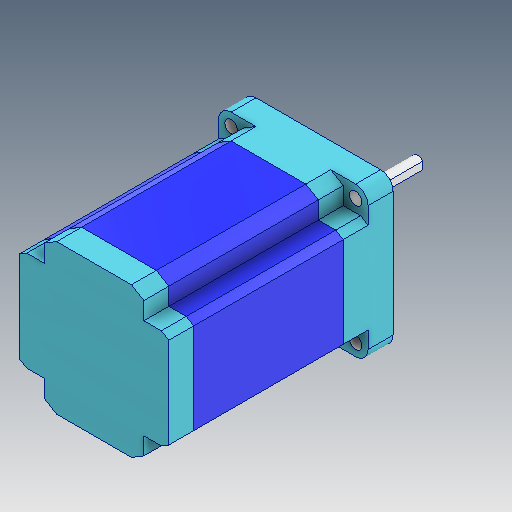
# Autodesk Inventor part: servo
Saved by Autodesk Inventor 2021 (Build 250183000, 183)
## iProperties
Created: 2021-07-07
Part Number: servo
Material: Generic
Document SubType Name: Modeling
Designer: Shaheen Khan
Density: 1 g/cm^3
Appearance: Aluminum - Flat
Author: Shaheen Khan
Autodesk Inventor part; units mm, degrees
ref_plane "XZ Plane" through (0, 0, 0) normal (0, 1, 0) x (-1, 0, 0)
ref_plane "XY Plane" through (0, 0, 0) normal (0, 0, 1) x (1, 0, 0)
sketch "Sketch1" plane through (0, 0, 0) normal (0, 0, 1) x (1, 0, 0)
  line L0 (-30, 30) -> (30, 30)
  line L1 (30, 30) -> (30, -30)
  line L2 (30, -30) -> (-30, -30)
  line L3 (-30, -30) -> (-30, 30)
  line L4 (-30, 30) -> (30, -30) construction
  line L5 (30, 30) -> (-30, -30) construction
  point P0 (0, 0)
  dimension "d0" = 60
  dimension "d1" = 60
  constraints: 12 end point, 2 midpoint, 2 parallel, 1 horizontal, 1 perpendicular
  measures "d0" distance of L1.end L2.end
  measures "d1" distance of L0.end L1.end
extrude "Extrusion1" add sketch "Sketch1" along normal blind 10
sketch "Sketch2" plane through (0, 0, 10) normal (0, 0, 1) x (1, 0, 0)
  line L0 (-30, -30) -> (30, -30) projected
  line L1 (30, -30) -> (30, 30) projected
  line L2 (30, 30) -> (-30, 30) projected
  line L3 (-30, 30) -> (-30, -30) projected
  line L4 (30, 30) -> (-30, 30) projected
  line L5 (0, 30) -> (-15, 30)
  line L6 (-15, 30) -> (-20, 27)
  line L7 (-20, 27) -> (-20, 20)
  line L8 (-20, 20) -> (-27, 20)
  line L9 (-27, 20) -> (-30, 18.2)
  line L10 (-30, 30) -> (-30, -30) projected
  line L11 (0, 30) -> (0, 0)
  line L12 (0, 0) -> (-30, 0)
  line L13 (15, 30) -> (20, 27)
  line L14 (20, 27) -> (20, 20)
  line L15 (20, 20) -> (27, 20)
  line L16 (27, 20) -> (30, 18.2)
  line L17 (0, -30) -> (-15, -30)
  line L18 (-15, -30) -> (-20, -27)
  line L19 (-20, -27) -> (-20, -20)
  line L20 (-20, -20) -> (-27, -20)
  line L21 (-27, -20) -> (-30, -18.2)
  line L22 (15, -30) -> (20, -27)
  line L23 (20, -27) -> (20, -20)
  line L24 (20, -20) -> (27, -20)
  line L25 (27, -20) -> (30, -18.2)
  dimension "d4" = 15
  dimension "d5" = 3
  dimension "d6" = 5
  dimension "d7" = 10
  dimension "d8" = 3
  constraints: 40 end point, 16 symmetric about line, 2 midpoint, 2 perpendicular, 2 point on line, 1 parallel
  measures "d4" distance of L5.start L5.end
  measures "d5" vertical distance of L6.end L5.end
  measures "d6" horizontal distance of L5.end L6.end
  measures "d7" distance between parallel lines of L8 L2
  measures "d8" horizontal distance of L8.end L9.end
extrude "Extrusion2" add sketch "Sketch2" along normal blind 10 contours L18 L19 L20 L21 L3 L12 L11 L2 L13 L14 L15 L16 L1 L25 L24 L23 L22 L0 | L3 L9 L8 L7 L6 L2 L11 L12
sketch "Sketch3" plane through (0, 0, 20) normal (0, 0, 1) x (1, 0, 0)
  line L0 (-27, 20) -> (-30, 18.2) projected
  line L1 (-30, 18.2) -> (-30, -18.2) projected
  line L2 (-30, -18.2) -> (-27, -20) projected
  line L3 (-27, -20) -> (-20, -20) projected
  line L4 (-20, -20) -> (-20, -27) projected
  line L5 (-20, -27) -> (-15, -30) projected
  line L6 (-15, -30) -> (15, -30) projected
  line L7 (15, -30) -> (20, -27) projected
  line L8 (20, -27) -> (20, -20) projected
  line L9 (20, -20) -> (27, -20) projected
  line L10 (27, -20) -> (30, -18.2) projected
  line L11 (30, -18.2) -> (30, 18.2) projected
  line L12 (30, 18.2) -> (27, 20) projected
  line L13 (27, 20) -> (20, 20) projected
  line L14 (20, 20) -> (20, 27) projected
  line L15 (20, 27) -> (15, 30) projected
  line L16 (15, 30) -> (-15, 30) projected
  line L17 (-15, 30) -> (-20, 27) projected
  line L18 (-20, 27) -> (-20, 20) projected
  line L19 (-20, 20) -> (-27, 20) projected
  point P0 (0, 0)
extrude "Extrusion3" add sketch "Sketch3" along normal blind 60 separate body
sketch "Sketch4" plane through (0, 0, 80) normal (0, 0, 1) x (1, 0, 0)
  line L0 (-30, 18.2) -> (-30, -18.2) projected
  line L1 (-30, -18.2) -> (-27, -20) projected
  line L2 (-27, -20) -> (-20, -20) projected
  line L3 (-20, -20) -> (-20, -27) projected
  line L4 (-20, -27) -> (-15, -30) projected
  line L5 (-15, -30) -> (15, -30) projected
  line L6 (15, -30) -> (20, -27) projected
  line L7 (20, -27) -> (20, -20) projected
  line L8 (20, -20) -> (27, -20) projected
  line L9 (27, -20) -> (30, -18.2) projected
  line L10 (30, -18.2) -> (30, 18.2) projected
  line L11 (30, 18.2) -> (27, 20) projected
  line L12 (27, 20) -> (20, 20) projected
  line L13 (20, 20) -> (20, 27) projected
  line L14 (20, 27) -> (15, 30) projected
  line L15 (15, 30) -> (-15, 30) projected
  line L16 (-15, 30) -> (-20, 27) projected
  line L17 (-20, 27) -> (-20, 20) projected
  line L18 (-20, 20) -> (-27, 20) projected
  line L19 (-27, 20) -> (-30, 18.2) projected
  point P0 (0, 0)
extrude "Extrusion4" add sketch "Sketch4" along normal blind 10 separate body
fillet "Fillet1" radius 5 4 edges at (30, 30, 5) (30, -30, 5) (-30, 30, 5) (-30, -30, 5)
sketch "Sketch5" plane through (0, 0, 0) normal (0, 0, -1) x (-1, 0, 0)
  line L0 (-25, -25) -> (25, -25) construction
  line L1 (25, -25) -> (25, 25) construction
  line L2 (25, 25) -> (-25, 25) construction
  line L3 (-25, 25) -> (-25, -25) construction
  line L4 (-25, -25) -> (25, 25) construction
  line L5 (25, -25) -> (-25, 25) construction
  point P0 (0, 0)
  dimension "d16" = 50
  dimension "d17" = 50
  constraints: 12 end point, 2 midpoint, 2 parallel, 1 horizontal, 1 perpendicular
  measures "d16" distance of L2.end L1.end
  measures "d17" distance of L1.end L0.end
hole "Hole1" at (-25, 25, 0) at (-25, -25, 0) at (25, 25, 0) at (25, -25, 0) direction (0, 0, 1) diameter 5 end through all bodies 1
sketch "Sketch6" plane through (0, 0, 0) normal (0, 0, -1) x (-1, 0, 0)
  circle A0 centre (0, 0) radius 20
  circle A1 centre (0, 0) radius 18
  dimension "d25" = 40
  dimension "d26" = 36
  constraints: 2 centre point, 2 coincident
  measures "d25" diameter of A0
  measures "d26" diameter of A1
extrude "Extrusion5" cut sketch "Sketch6" against normal blind 0.5 bodies 1
sketch "Sketch7" plane through (0, 0, 0) normal (0, 0, -1) x (-1, 0, 0)
  circle A0 centre (0, 0) radius 2.5
  line L0 (-6, -2) -> (6, -2)
  line L1 (6, -2) -> (6, 2)
  line L2 (6, 2) -> (-6, 2)
  line L3 (-6, 2) -> (-6, -2)
  line L4 (-6, -2) -> (6, 2) construction
  line L5 (6, -2) -> (-6, 2) construction
  line L6 (-2, -6) -> (2, -6)
  line L7 (2, -6) -> (2, 6)
  line L8 (2, 6) -> (-2, 6)
  line L9 (-2, 6) -> (-2, -6)
  line L10 (-2, -6) -> (2, 6) construction
  line L11 (2, -6) -> (-2, 6) construction
  point P0 (2, 2)
  point P1 (-2, 2)
  point P2 (-2, -2)
  point P3 (2, -2)
  dimension "d29" = 5
  dimension "d30" = 12
  dimension "d31" = 4
  dimension "d32" = 4
  dimension "d33" = 12
  constraints: 24 end point, 4 midpoint, 4 parallel, 2 horizontal, 2 perpendicular, 1 centre point, 1 coincident
  measures "d29" diameter of A0
  measures "d30" distance of L2.end L1.end
  measures "d31" distance of L1.end L0.end
  measures "d32" distance of L8.end L7.end
  measures "d33" distance of L7.end L6.end
extrude "Extrusion6" cut sketch "Sketch7" against normal through all bodies 1
sketch "Sketch8" plane through (0, 0, 0) normal (0, 0, -1) x (-1, 0, 0)
  circle A0 centre (0, 0) radius 2.5
  dimension "d36" = 5
  constraints: 1 centre point, 1 coincident
  measures "d36" diameter of A0
extrude "Extrusion7" add sketch "Sketch8" along normal blind 40 bodies 1
sketch "Sketch9" plane through (0, 0, -40) normal (0, 0, -1) x (-1, 0, 0)
  circle A0 centre (0, 0) radius 2.5 projected
  line L0 (-2, 1.5) -> (-2, -1.5)
  dimension "d39" = 2
  constraints: 2 end point, 2 point on circle, 1 vertical
  measures "d39" distance from line of L0 point (0, 0)
extrude "Extrusion8" cut sketch "Sketch9" against normal blind 15 contours L0 A0 picked at (-2.0912, -0.3466) bodies 1
sketch "Sketch10" plane through (0, 0, -40) normal (0, 0, -1) x (-1, 0, 0)
  circle A0 centre (0, 0) radius 2.5 projected
  constraints: 1 coincident
hole "Hole2" at (0, 0, -40) direction (0, 0, 1) diameter 0.5 end through all countersink diameter 2.5 countersink angle 90 bodies 1
sketch "Sketch11" plane through (0, 0, 0) normal (0, 0, -1) x (-1, 0, 0)
  circle A0 centre (0, 0) radius 2.5 projected
  arc A1 (3.7749, -14) -> (14, -3.7749) centre (0, 0) ccw construction
  arc A2 (4.2956, -15.931) -> (15.931, -4.2956) centre (0, 0) ccw
  arc A3 (3.2542, -12.069) -> (12.069, -3.2542) centre (0, 0) ccw
  arc A4 (3.2542, -12.069) -> (4.2956, -15.931) centre (3.7749, -14) ccw
  arc A5 (15.931, -4.2956) -> (12.069, -3.2542) centre (14, -3.7749) ccw
  dimension "d49" = 14.5
  dimension "d50" = 14
  dimension "d51" = 14
  dimension "d52" = 2
  constraints: 10 point on circle, 5 centre point, 4 tangent, 1 coincident
  measures "d49" radius of A1
  measures "d50" horizontal distance of point (0, 0) A1.end
  measures "d51" vertical distance of A1.start point (0, 0)
  measures "d52" radius of A4
extrude "Extrusion9" cut sketch "Sketch11" against normal blind 0.5 contours A4 A3 A5 A2 bodies 1
pattern_circular "Circular Pattern1" count 4 over 360 about axis through (0, 0, 0) along (0, 0, 1) of "Extrusion9" bodies 1
ref_plane "Work Plane1" through (0, 0, 0) normal (1, 0, 0) x (0, 1, 0)
body "Solid1"
body "Solid2"
body "Solid3"
